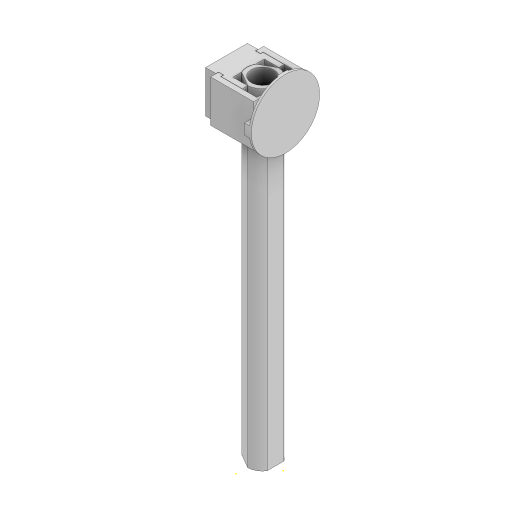
# Autodesk Inventor part: Funda_Escoba_v1
Saved by Autodesk Inventor 2024 (Build 280153000, 153)
## iProperties
Created: 2023-10-21
Part Number: Funda_Escoba_v1
Material: Generic
Document SubType Name: Modeling
Designer: Alvaromf6
Density: 1 g/cm^3
Appearance: Default
Author: Alvaromf6
Autodesk Inventor part; units mm, degrees
ref_plane "YZ Plane" through (0, 0, 0) normal (1, 0, 0) x (0, 1, 0)
ref_plane "XZ Plane" through (0, 0, 0) normal (0, 1, 0) x (-1, 0, 0)
ref_plane "XY Plane" through (0, 0, 0) normal (0, 0, 1) x (1, 0, 0)
sketch "Sketch1" plane through (0, 0, 0) normal (0, 1, 0) x (-1, 0, 0)
  circle A0 centre (0, 0) radius 10.765
  line L0 (0, 0) -> (162.1519, 0) construction
  line L1 (0, 0) -> (190.4731, 0) construction
  line L2 (0, 0) -> (10.765, 0) construction
  line L3 (6.1825, -10.7084) -> (13.1107, -6.7084)
  line L4 (6.1825, -10.7084) -> (-0.7457, -14.7084)
  line L5 (6.1825, 10.7084) -> (-0.7457, 14.7084)
  line L6 (6.1825, 10.7084) -> (13.1107, 6.7084)
  line L7 (-12.365, 0) -> (-12.365, -8)
  line L8 (-12.365, 0) -> (-12.365, 8)
  arc A1 (-0.7457, 14.7084) -> (-12.365, 8) centre (0, 0) ccw
  arc A2 (-12.365, -8) -> (-0.7457, -14.7084) centre (0, 0) ccw
  arc A3 (13.1107, -6.7084) -> (13.1107, 6.7084) centre (0, 0) ccw
  dimension "d6" = 8
  dimension "d7" = 8
  dimension "d8" = 21.53
  dimension "d11" = 360
  constraints: 18 end point, 6 point on circle, 4 centre point, 3 horizontal, 3 point on line, 2 coincident, 16 other
  measures "d6" distance of L3.start L3.end
  measures "d7" distance of L3.start L4.end
  measures "d8" diameter of A0
extrude "Extrusion1" add sketch "Sketch1" along normal blind 315
sketch "Sketch2" plane through (0, 315, 0) normal (0, 1, 0) x (1, 0, 0)
  arc A0 (-13.1107, 6.7084) -> (-13.1107, -6.7084) centre (0, 0) ccw projected
  arc A1 (-13.2887, 6.7995) -> (-13.2887, -6.7995) centre (0, 0) ccw
  line L0 (-13.2887, 6.7995) -> (-13.2887, 14.9584)
  line L1 (0.7457, 14.9584) -> (-13.2887, 14.9584)
  circle A2 centre (0, 0) radius 10.765 projected
  line L2 (-13.2887, -6.7995) -> (-13.2887, -14.9584)
  line L3 (0.7457, -14.9584) -> (-13.2887, -14.9584)
  line L4 (0.7457, 14.9584) -> (0.7457, 19.9584)
  line L5 (-34.2543, 19.9584) -> (-34.2543, 0)
  line L6 (0.7457, -14.9584) -> (0.7457, -19.9584)
  line L7 (-34.2543, -19.9584) -> (-34.2543, 0)
  line L8 (-19.3823, 19.9584) -> (-19.3823, 17.4584)
  line L9 (-19.3823, 17.4584) -> (-24.3823, 17.4584)
  line L10 (-24.3823, 17.4584) -> (-24.3823, 19.9584)
  line L11 (0.7457, 19.9584) -> (-19.3823, 19.9584)
  line L12 (-24.3823, 19.9584) -> (-34.2543, 19.9584)
  line L13 (-19.3823, -19.9584) -> (-19.3823, -17.4584)
  line L14 (-19.3823, -17.4584) -> (-24.3823, -17.4584)
  line L15 (-24.3823, -17.4584) -> (-24.3823, -19.9584)
  line L16 (0.7457, -19.9584) -> (-19.3823, -19.9584)
  line L17 (-24.3823, -19.9584) -> (-34.2543, -19.9584)
  dimension "d15" = 0.2
  dimension "d18" = 5
  dimension "d19" = 35
  dimension "d20" = 5
  constraints: 36 end point, 8 perpendicular, 3 vertical, 2 point on circle, 1 centre point
  measures "d15" radial gap between concentric circles of A0 A1
  measures "d18" distance of L1.start L4.end
  measures "d19" distance of L4.end L5.start
  measures "d20" distance of L8.end L9.end
extrude "Extrusion2" add sketch "Sketch2" against normal blind 40 separate body contours A1 L2 L3 L6 L16 L13 L14 L15 L17 L7 L5 L12 L10 L9 L8 L11 L4 L1 L0
sketch "Sketch3" plane through (0, 315, 0) normal (0, 1, 0) x (1, 0, 0)
  line L0 (-19.3823, 19.9584) -> (-19.3823, 17.4584) projected
  line L1 (-19.3823, 17.4584) -> (-24.3823, 17.4584) projected
  line L2 (-24.3823, 17.4584) -> (-24.3823, 19.9584) projected
  line L3 (-19.6323, 19.9584) -> (-19.6323, 17.7084)
  line L4 (-19.6323, 17.7084) -> (-24.1323, 17.7084)
  line L5 (-24.1323, 17.7084) -> (-24.1323, 19.9584)
  line L6 (-19.6323, 19.9584) -> (-19.6323, 20.2084)
  line L7 (-19.3823, 19.9584) -> (0.7457, 19.9584) projected
  line L8 (-19.6323, 19.9584) -> (-19.3823, 19.9584) construction
  line L9 (-19.6323, 20.2084) -> (14.865, 20.2084)
  line L10 (12.365, -8) -> (12.365, 8) projected
  line L11 (12.365, 0) -> (14.865, 0)
  line L12 (14.865, 0) -> (14.865, 20.2084)
  line L13 (-24.1323, 19.9584) -> (-24.1323, 25.2084)
  line L14 (-24.1323, 25.2084) -> (14.865, 25.2084)
  line L15 (14.865, 25.2084) -> (16.865, 25.2084)
  line L16 (16.865, 25.2084) -> (16.865, 0)
  line L17 (0, 0) -> (2.9179, 0)
  line L18 (-19.6323, -19.9584) -> (-19.6323, -17.7084)
  line L19 (-19.6323, -17.7084) -> (-24.1323, -17.7084)
  line L20 (-24.1323, -17.7084) -> (-24.1323, -19.9584)
  line L21 (-19.6323, -19.9584) -> (-19.6323, -20.2084)
  line L22 (-19.3823, -19.9584) -> (0.7457, -19.9584)
  line L23 (-19.6323, -19.9584) -> (-19.3823, -19.9584) construction
  line L24 (-19.6323, -20.2084) -> (14.865, -20.2084)
  line L25 (14.865, 0) -> (14.865, -20.2084)
  line L26 (-24.1323, -19.9584) -> (-24.1323, -25.2084)
  line L27 (-24.1323, -25.2084) -> (14.865, -25.2084)
  line L28 (14.865, -25.2084) -> (16.865, -25.2084)
  line L29 (16.865, -25.2084) -> (16.865, 0)
  point P0 (-19.3823, -17.4584)
  dimension "d23" = 0.25
  dimension "d24" = 0.25
  dimension "d25" = 90
  dimension "d26" = 90
  dimension "d27" = 2.5
  dimension "d28" = 5.25
  dimension "d29" = 2
  constraints: 50 end point, 13 symmetric about line, 5 perpendicular, 4 horizontal, 2 point on line, 1 midpoint, 1 parallel, 2 other
  measures "d23" distance between parallel lines of L0 L3
  measures "d24" distance of L3.start L6.end
  measures "d25" angle of L8 L6
  measures "d26" angle of L6 L9
  measures "d27" distance of L11.start L11.end
  measures "d28" distance of L5.end L13.end
  measures "d29" distance of L14.end L15.end
extrude "Extrusion3" add sketch "Sketch3" against normal blind 40 separate body
sketch "Sketch4" plane through (16.865, 315, 25.2084) normal (1, 0, 0) x (0, 0, -1)
  line L0 (33.2084, -315) -> (33.2084, 0) projected
  line L1 (17.2084, -315) -> (17.2084, 0) projected
  line L2 (0, 0) -> (0, -40) projected
  line L3 (0, 0) -> (50.4168, 0) projected
  line L4 (50.4168, 0) -> (50.4168, -40) projected
  line L5 (50.4168, -40) -> (0, -40) projected
  line L6 (27.9584, -22.75) -> (22.4584, -22.75)
  line L7 (22.4584, -22.75) -> (22.4584, -17.25)
  line L8 (22.4584, -17.25) -> (27.9584, -17.25)
  line L9 (27.9584, -17.25) -> (27.9584, -22.75)
  line L10 (27.9584, -22.75) -> (22.4584, -17.25) construction
  line L11 (22.4584, -22.75) -> (27.9584, -17.25) construction
  point P0 (25.2084, -315)
  point P1 (25.2084, -20)
  dimension "d32" = 5.5
  dimension "d33" = 5.5
  constraints: 12 end point, 2 midpoint, 2 parallel, 1 horizontal, 1 perpendicular
  measures "d32" distance of L7.end L8.end
  measures "d33" distance of L6.end L7.end
extrude "Extrusion4" cut sketch "Sketch4" against normal blind 3.4875 contours L6 L7 L8 L9 bodies 3
sketch "Sketch5" plane through (16.865, 315, 25.2084) normal (1, 0, 0) x (0, 0, -1)
  line L0 (22.4584, -22.75) -> (22.4584, -17.25) projected
  line L1 (27.9584, -22.75) -> (22.4584, -22.75) projected
  line L2 (27.9584, -17.25) -> (27.9584, -22.75) projected
  line L3 (22.4584, -17.25) -> (27.9584, -17.25) projected
  line L4 (27.7084, -17.5) -> (27.7084, -22.5)
  line L5 (27.7084, -22.5) -> (22.7084, -22.5)
  line L6 (22.7084, -22.5) -> (22.7084, -17.5)
  line L7 (22.7084, -17.5) -> (27.7084, -17.5)
  point P0 (25.2084, -315)
  dimension "d36" = 0.25
  constraints: 8 end point, 3 other
  measures "d36" distance between parallel lines of L3 L7
extrude "Extrusion5" add sketch "Sketch5" along normal mid plane 6 separate body contours L4 L5 L6 L7
sketch "Sketch6" plane through (19.865, 315, 25.2084) normal (1, 0, 0) x (0, 0, -1)
  line L0 (27.7084, -22.5) -> (27.7084, -17.5) projected
  line L1 (27.7084, -17.5) -> (22.7084, -17.5) projected
  line L2 (22.7084, -17.5) -> (22.7084, -22.5) projected
  line L3 (22.7084, -22.5) -> (27.7084, -22.5) projected
  line L4 (22.7084, -17.5) -> (22.7084, -22.5) projected
  line L5 (22.7084, -22.5) -> (27.7084, -22.5) projected
  line L6 (27.7084, -22.5) -> (27.7084, -17.5) projected
  line L7 (27.7084, -17.5) -> (22.7084, -17.5) projected
  circle A0 centre (25.2084, -20) radius 32.5
  point P0 (25.2084, -315)
  dimension "d39" = 65
  constraints: 1 centre point
  measures "d39" diameter of A0
extrude "Extrusion6" add sketch "Sketch6" along normal blind 2 bodies 4
sketch "Sketch7" plane through (19.865, 315, 25.2084) normal (1, 0, 0) x (0, 0, -1)
  point P0 (25.2084, -315)
sketch "Sketch8" plane through (21.865, 295, 0) normal (1, 0, 0) x (0, 0, -1)
  line L0 (-2.5, -2.5) -> (-2.5, 2.5) projected
  line L1 (-2.5, 2.5) -> (2.5, 2.5) projected
  line L2 (2.5, 2.5) -> (2.5, -2.5) projected
  line L3 (2.5, -2.5) -> (-2.5, -2.5) projected
  point P0 (0, -295)
extrude "Extrusion7" add sketch "Sketch8" against normal blind 2.35 bodies 4
sketch "Sketch9" plane through (13.865, 315, 25.2084) normal (-1, 0, 0) x (0, 0, 1)
  line L0 (-29.608, -15.5608) -> (-20.4879, -15.5608)
  line L1 (-20.4879, -15.5608) -> (-20.4879, -24.3637)
  line L2 (-20.4879, -24.3637) -> (-29.608, -24.3637)
  line L3 (-29.608, -24.3637) -> (-29.608, -15.5608)
  point P0 (-25.2084, -315)
  constraints: 8 end point, 2 parallel, 1 horizontal, 1 perpendicular
extrude "Extrusion8" cut sketch "Sketch9" against normal blind 3.0875 bodies 4
sketch "Sketch10" plane through (19.865, 295, 0) normal (-1, 0, 0) x (0, 0, 1)
  line L0 (-2.5, 2.5) -> (2.5, 2.5) projected
  line L1 (-2.5, -2.5) -> (-2.5, 2.5) projected
  line L2 (2.5, -2.5) -> (-2.5, -2.5) projected
  line L3 (2.5, 2.5) -> (2.5, -2.5) projected
  line L4 (-2.25, -2.25) -> (2.25, -2.25)
  line L5 (2.25, -2.25) -> (2.25, 2.25)
  line L6 (2.25, 2.25) -> (-2.25, 2.25)
  line L7 (-2.25, 2.25) -> (-2.25, -2.25)
  line L8 (-2.25, -2.25) -> (2.25, 2.25) construction
  line L9 (2.25, -2.25) -> (-2.25, 2.25) construction
  line L10 (-2.5, 2.5) -> (2.5, 2.5)
  line L11 (2.5, 2.5) -> (2.5, -2.5)
  line L12 (2.5, -2.5) -> (-2.5, -2.5)
  line L13 (-2.5, -2.5) -> (-2.5, 2.5)
  line L14 (-2.5, 2.5) -> (2.5, -2.5) construction
  line L15 (2.5, 2.5) -> (-2.5, -2.5) construction
  point P0 (0, -295)
  point P1 (0, 0)
  dimension "d46" = 4.5
  dimension "d47" = 4.5
  constraints: 24 end point, 4 midpoint, 4 parallel, 2 horizontal, 2 perpendicular
  measures "d46" distance of L6.end L5.end
  measures "d47" distance of L5.end L4.end
extrude "Extrusion9" cut sketch "Sketch10" along normal blind 6.2625 bodies 4
sketch "Sketch11" plane through (-24.1323, 315, 25.2084) normal (0, 0, 1) x (1, 0, 0)
  point P0 (24.1323, -315)
sketch "Sketch12" plane through (19.865, 295, 0) normal (-1, 0, 0) x (0, 0, 1)
  circle A0 centre (0, 0) radius 32.5 projected
  line L0 (25.2084, 20) -> (25.2084, -20) projected
  line L1 (25.4, 0) -> (25.4, 5)
  line L2 (25.4, 5) -> (32.1131, 5)
  arc A1 (32.5, 0) -> (32.1131, 5) centre (0, 0) ccw
  line L3 (25.4, 0) -> (25.4, -5)
  line L4 (25.4, -5) -> (32.1131, -5)
  arc A2 (32.1131, -5) -> (32.5, 0) centre (0, 0) ccw
  line L5 (-25.4, 0) -> (-25.4, 5)
  line L6 (-25.4, 5) -> (-32.1131, 5)
  arc A3 (-32.1131, 5) -> (-32.5, 0) centre (0, 0) ccw
  line L7 (-25.4, -5) -> (-32.1131, -5)
  line L8 (-25.4, 0) -> (-25.4, -5)
  arc A4 (-32.5, 0) -> (-32.1131, -5) centre (0, 0) ccw
  point P0 (0, -295)
  point P1 (32.1131, -5)
  point P2 (-32.1131, 5)
  point P3 (-32.1131, -5)
  dimension "d50" = 7.1
  dimension "d52" = 5
  constraints: 16 end point, 10 point on circle, 4 centre point, 1 concentric, 1 horizontal, 1 vertical
  measures "d50" distance of A0.start L1.start
  measures "d52" distance of L1.start L1.end
extrude "Extrusion10" add sketch "Sketch12" along normal blind 5 contours A0 L4 L3 L1 L2 | L6 L5 L8 L7 A0 bodies 4
sketch "Sketch13" plane through (19.865, 315, 25.2084) normal (-1, 0, 0) x (0, 0, 1)
  line L0 (-18.5, 0) -> (-31.9168, 0) projected
  line L1 (-25.2084, 0.25) -> (-20.2084, 0.25)
  arc A0 (6.9047, -15) -> (-57.3215, -15) centre (-25.2084, -20) ccw projected
  line L2 (-20.2084, 0.25) -> (-20.2084, 12.1131)
  line L3 (-25.2084, 0.25) -> (-30.2084, 0.25)
  line L4 (-30.2084, 0.25) -> (-30.2084, 12.1131)
  arc A1 (-20.2084, 12.1131) -> (-30.2084, 12.1131) centre (-25.2084, -20) ccw
  line L5 (-25.2084, -40.25) -> (-20.2084, -40.25)
  line L6 (-20.2084, -40.25) -> (-20.2084, -52.1131)
  line L7 (-25.2084, -40.25) -> (-30.2084, -40.25)
  line L8 (-30.2084, -40.25) -> (-30.2084, -52.1131)
  arc A2 (-30.2084, -52.1131) -> (-20.2084, -52.1131) centre (-25.2084, -20) ccw
  point P0 (-25.2084, -315)
  point P1 (-18.5, -40)
  dimension "d56" = 5
  dimension "d57" = 5
  constraints: 16 end point, 6 point on circle, 2 centre point, 2 perpendicular, 1 vertical
  measures "d56" distance of L1.start L1.end
  measures "d57" distance of L1.start L3.end
extrude "Extrusion11" add sketch "Sketch13" along normal blind 5 bodies 4
sketch "Sketch14" plane through (14.865, 315, 25.2084) normal (-1, 0, 0) x (0, 0, 1)
  line L0 (-20.2084, 0.25) -> (-20.2084, 0.3)
  line L1 (-20.2084, 0.25) -> (-20.2084, 12.1131) projected
  line L2 (-30.2084, 0.3) -> (-50.6584, 0.3)
  line L3 (-50.6084, -15) -> (-50.6084, -25) projected
  line L4 (-50.6084, -15) -> (-50.6584, -15)
  line L5 (-50.6584, -15) -> (-50.6584, 0.3)
  line L6 (-30.2084, 0.3) -> (-25.2084, 0.3)
  line L7 (-50.6584, -15) -> (-50.6584, -20)
  line L8 (-20.2084, 0.3) -> (0.2416, 0.3)
  line L9 (0.1916, -15) -> (0.2416, -15)
  line L10 (0.2416, -15) -> (0.2416, 0.3)
  line L11 (-20.2084, 0.3) -> (-25.2084, 0.3)
  line L12 (0.2416, -15) -> (0.2416, -20)
  line L13 (-20.2084, -40.25) -> (-20.2084, -40.3)
  line L14 (-30.2084, -40.3) -> (-50.6584, -40.3)
  line L15 (-50.6584, -25) -> (-50.6584, -40.3)
  line L16 (-30.2084, -40.3) -> (-25.2084, -40.3)
  line L17 (-50.6584, -25) -> (-50.6584, -20)
  line L18 (-20.2084, -40.3) -> (0.2416, -40.3)
  line L19 (0.2416, -25) -> (0.2416, -40.3)
  line L20 (0.2416, -25) -> (0.2416, -20)
  line L21 (-20.2084, -40.3) -> (-25.2084, -40.3)
  line L22 (-29.4997, -16.0212) -> (-20.2084, -16.0212)
  line L23 (-20.2084, -16.0212) -> (-20.2084, -24.0433)
  line L24 (-20.2084, -24.0433) -> (-29.4997, -24.0433)
  line L25 (-29.4997, -24.0433) -> (-29.4997, -16.0212)
  point P0 (-25.2084, -315)
  point P1 (6.9047, -15)
  dimension "d60" = 0.05
  dimension "d61" = 0.05
  constraints: 48 end point, 3 perpendicular, 2 parallel, 1 horizontal, 1 point on line
  measures "d60" distance of L0.start L0.end
  measures "d61" distance of L3.start L4.end
extrude "Extrusion12" cut sketch "Sketch14" against normal blind 5 bodies 4
sketch "Sketch15" plane through (14.865, 295, 0) normal (-1, 0, 0) x (0, 0, 1)
  line L0 (-12.8519, 40.0431) -> (11.8192, 40.0431)
  line L1 (11.8192, 40.0431) -> (11.8192, 16.7136)
  line L2 (11.8192, 16.7136) -> (-12.8519, 16.7136)
  line L3 (-12.8519, 16.7136) -> (-12.8519, 40.0431)
  line L4 (-18.8893, -12.8023) -> (17.1858, -12.8023)
  line L5 (17.1858, -12.8023) -> (17.1858, -35.3865)
  line L6 (17.1858, -35.3865) -> (-18.8893, -35.3865)
  line L7 (-18.8893, -35.3865) -> (-18.8893, -12.8023)
  point P0 (0, -295)
  constraints: 16 end point, 4 parallel, 2 horizontal, 2 perpendicular
extrude "Extrusion13" cut sketch "Sketch15" against normal blind 4 bodies 4
body "Solid1"
body "Solid2"
body "Solid3"
body "Solid4"
